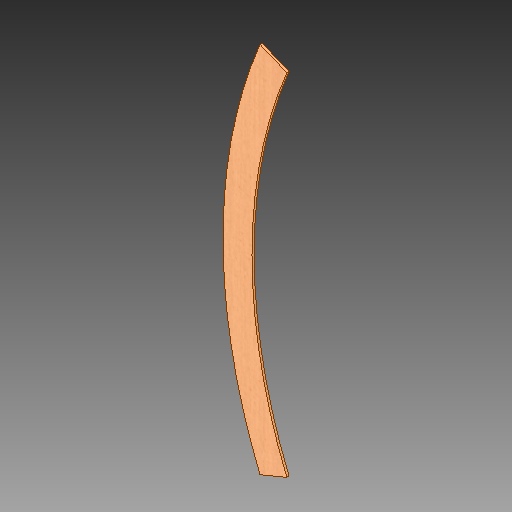
# Autodesk Inventor part: rearformer3
Saved by Autodesk Inventor 2019 (Build 230136000, 136)
## iProperties
Created: 2019-01-07
Part Number: rearformer3
Material: Wood (Cherry)
Document SubType Name: Modeling
Designer: gaincarlo
Density: 0.63 g/cm^3
Appearance: Cherry - Natural Low Gloss
Author: gaincarlo
Autodesk Inventor part; units mm, degrees
ref_plane "YZ Plane" through (0, 0, 0) normal (1, 0, 0) x (0, 1, 0)
ref_plane "XZ Plane" through (0, 0, 0) normal (0, 1, 0) x (-1, 0, 0)
ref_plane "Work Plane1" through (0, 0, 450) normal (0, 0, 1) x (1, 0, 0)
sketch "Sketch1" plane through (0, 0, 450) normal (0, 0, 1) x (1, 0, 0)
  line L0 (-254.3277, 283.4578) -> (-250.5009, 292.6966) construction
  line L1 (-250.5009, 292.6966) -> (303.8268, 63.0866) construction
  line L2 (303.8268, 63.0866) -> (300, 53.8478) construction
  line L3 (300, 53.8478) -> (-254.3277, 283.4578) construction
  line L4 (300, -53.8478) -> (303.8268, -63.0866) construction
  line L5 (303.8268, -63.0866) -> (-250.5009, -292.6966) construction
  line L6 (-250.5009, -292.6966) -> (-254.3277, -283.4578) construction
  line L7 (-254.3277, -283.4578) -> (300, -53.8478) construction
  arc A0 (-152.3888, 239.0623) -> (-152.3888, -239.0623) centre (430, 0) ccw construction
  spline S0 degree 3 poles (-152.3888, -239.0623) (-152.7274, -239.2015) (-153.0661, -239.3407) (-153.7434, -239.6192) (-154.082, -239.7584) (-154.4207, -239.8976) knots -0.219692 -0.219692 -0.219692 -0.219692 -0.109846 -0.109846 0 0 0 0 construction
  arc A1 (-154.4207, 239.8976) -> (-154.4207, -239.8976) centre (430, 0) ccw construction
  spline S1 degree 3 poles (-154.4207, 239.8976) (-154.082, 239.7584) (-153.7434, 239.6192) (-153.0661, 239.3407) (-152.7274, 239.2015) (-152.3888, 239.0623) knots -0.219692 -0.219692 -0.219692 -0.219692 -0.109846 -0.109846 0 0 0 0 construction
  line L8 (-190.609, 257.0647) -> (-153.6538, 241.7573)
  line L9 (-190.609, -257.0647) -> (-153.6538, -241.7573)
  arc A2 (-153.6538, 241.7573) -> (-153.6538, -241.7573) centre (430, 0) ccw
  arc A3 (-190.609, 257.0647) -> (-190.609, -257.0647) centre (430, 0) ccw
  point P0 (0, 0)
  dimension "d3" = 40
  constraints: 20 end point, 8 point on circle, 4 centre point, 4 point on line, 2 coincident, 30 other
  measures "d3" radial gap between concentric circles of A3 A1
extrude "Extrusion1" add sketch "Sketch1" against normal blind 3
body "Solid1"
